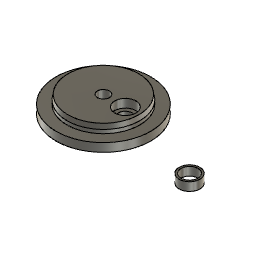
connector cap v26 (Autodesk Fusion 360 design; units mm, degrees)
Autodesk Fusion 360 part; units mm, degrees
sketch "Sketch7" plane through (0, 0, 0) normal (0, 0, 1) x (1, 0, 0)
  circle A0 centre (0, 0) radius 28
  dimension "d21" = 56
  constraint coincident A0.centre origin
  measures "d21" diameter of A0
extrude "Extrude7" add sketch "Sketch7" along normal blind 20 makes body 1
sketch "Sketch8" plane through (0, 0, 20) normal (0, 0, 1) x (-1, 0, 0)
  circle A0 centre (0, 0) radius 28
  circle A1 centre (0, 0) radius 21
  dimension "d24" = 42
  constraint coincident A0.centre A1.centre
  measures "d24" diameter of A1
extrude "Extrude8" cut sketch "Sketch8" against normal blind 5 bodies 1
sketch "Sketch9" plane through (0, 0, 0) normal (0, 0, -1) x (1, 0, 0)
  circle A0 centre (0, 0) radius 28
  circle A1 centre (0, 0) radius 5
  circle A2 centre (13, 0) radius 6.25
  dimension "d27" = 10
  dimension "d28" = 12.5
  constraint coincident A0.centre A1.centre
  measures "d27" diameter of A1
  measures "d28" diameter of A2
extrude "Extrude9" cut sketch "Sketch9" against normal blind 20 contours A1 | A2 bodies 1
extrude "Extrude10" cut 1 faces at (5.7394, 12.5284, 0) along direction (0, 0, 1) blind 10 on bodies 1 bodies 1
extrude "Extrude11" add 1 faces at (5.7394, 12.5284, 10) along direction (0, 0, -1) blind 5 on bodies 1 bodies 1
sketch "Sketch10" plane through (0, 0, 5) normal (0, 0, -1) x (1, 0, 0)
  circle A0 centre (0, 0) radius 5
  circle A1 centre (13, 0) radius 6.25
  circle A2 centre (0, 0) radius 28
  circle A3 centre (0, 0) radius 3
  dimension "d66" = 6
  constraint coincident A0.centre A2.centre
  measures "d66" diameter of A3
extrude "Extrude12" add sketch "Sketch10" against normal blind 5 contours A0 | A3 bodies 1
extrude "Extrude13" add 1 faces at (6.458, 9.8718, 20) along direction (0, 0, 1) blind 5 on bodies 1 bodies 1
extrude "Extrude14" cut 1 faces at (-16.3124, 1.3911, 5) along direction (0, 0, 1) blind 5 on bodies 1 bodies 1
sketch "Sketch11" plane through (0, 0, 10) normal (0, 0, -1) x (1, 0, 0)
  circle A0 centre (0, 0) radius 5
  circle A1 centre (13, 0) radius 6.25
  circle A2 centre (0, 0) radius 28
  circle A3 centre (0, 0) radius 5
  constraint concentric A0 A3
extrude "Extrude15" add sketch "Sketch11" against normal blind 5 contours A0 A3 bodies 1
sketch "Sketch12" plane through (0, 0, 10) normal (0, 0, -1) x (1, 0, 0)
  circle A0 centre (13, 0) radius 6.25
  circle A1 centre (0, 0) radius 28
  circle A2 centre (13, 0) radius 4
  constraint concentric A0 A2
extrude "Extrude16" add sketch "Sketch12" against normal blind 5 contours A0 bodies 1
sketch "Sketch13" plane through (0, 0, 0) normal (0, 0, 1) x (1, 0, 0)
  circle A0 centre (51, 0) radius 6.125
  circle A1 centre (51, 0) radius 5
  dimension "d45" = 12.25
  dimension "d46" = 10
  constraint concentric A0 A1
  measures "d45" diameter of A0
  measures "d46" diameter of A1
extrude "Extrude17" add sketch "Sketch13" along normal blind 10 separate body makes body 2
sketch "Sketch14" plane through (0, 0, 15) normal (0, 0, 1) x (-1, 0, 0)
  circle A0 centre (0, 0) radius 21
  circle A1 centre (0, 0) radius 28
  circle A2 centre (0, 0) radius 25.5
  dimension "d49" = 51
  constraint coincident A0.centre A1.centre
  measures "d49" diameter of A2
extrude "Extrude18" add sketch "Sketch14" along normal blind 5 contours A1 bodies 1
extrude "Extrude19" cut 1 faces at (6.458, 9.8718, 25) along direction (0, 0, -1) blind 5 on bodies 1 bodies 1
extrude "Extrude20" cut 1 faces at (56.7086, -0.5527, 10) along direction (0, 0, -1) blind 5 on bodies 2 bodies 2
sketch "Sketch15" plane through (0, 0, 20) normal (0, 0, 1) x (-1, 0, 0)
  circle A0 centre (-13, 0) radius 6.25
  circle A1 centre (0, 0) radius 21
  circle A2 centre (0, 0) radius 2.2856
  circle A3 centre (0, 0) radius 5
extrude "Extrude21" cut sketch "Sketch15" along normal blind 5 contours A3 bodies 1
sketch "Sketch19" plane through (0, 0, 20) normal (0, 0, 1) x (-1, 0, 0)
  circle A0 centre (0, 0) radius 5
  circle A1 centre (-13, 0) radius 6.25
  circle A2 centre (0, 0) radius 21
  circle A3 centre (0, 0) radius 21.5
  dimension "d74" = 0.5
extrude "Extrude26" add sketch "Sketch19" against normal blind 5 contours A3 bodies 1
extrude "Extrude22" cut 1 faces at (-27.0624, 1.3911, 20) along direction (0, 0, -1) blind 5 on bodies 1 bodies 1
sketch "Sketch16" plane through (0, 0, 10) normal (0, 0, -1) x (1, 0, 0)
  circle A0 centre (13, 0) radius 4
  circle A1 centre (0, 0) radius 28
  circle A2 centre (0, 0) radius 6.6395
  constraint coincident A1.centre A2.centre
  constraint concentric A1 A2
extrude "Extrude23" cut sketch "Sketch16" against normal blind 5 contours A2 bodies 1
sketch "Sketch17" plane through (0, 0, 20) normal (0, 0, 1) x (-1, 0, 0)
  circle A0 centre (-13, 0) radius 6.25
  circle A1 centre (0, 0) radius 5
  circle A2 centre (0, 0) radius 3.5
  circle A3 centre (0, 0) radius 21.5
  dimension "d69" = 7
  constraint concentric A1 A2
  measures "d69" diameter of A2
extrude "Extrude24" add sketch "Sketch17" against normal blind 5 contours A1 bodies 1
sketch "Sketch18" plane through (0, 0, 15) normal (0, 0, -1) x (1, 0, 0)
  circle A0 centre (0, 0) radius 3.5
  circle A1 centre (0, 0) radius 4
  circle A2 centre (0, 0) radius 5.5
  circle A3 centre (0, 0) radius 6.6395
  dimension "d70" = 8
  dimension "d71" = 11
  constraint concentric A0 A1
  constraint concentric A0 A2
  measures "d70" diameter of A1
  measures "d71" diameter of A2
extrude "Extrude25" cut sketch "Sketch18" against normal blind 0.5 contours A2 bodies 1
chamfer "Chamfer3" distance 0.5 angle 80 1 edges at (20.045, 7.7747, 20) measured on face at (4.8887, 9.7532, 20) on bodies 1
